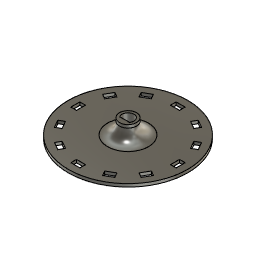
sterivex vortex adapter plate fusion360 (Autodesk Fusion 360 archive; units mm, degrees)
design "Untitled" references "jeej fixed mesh"
Autodesk Fusion 360 part; units mm, degrees
sketch "Sketch3" plane through (0, 0, 0) normal (0, 0, 1) x (1, 0, 0)
  circle A0 centre (0, 0) radius 80
  dimension "d8" = 160
  constraint coincident A0.centre origin
  measures "d8" diameter of A0
extrude "Extrude3" add sketch "Sketch3" along normal blind 4 makes body 1
sketch "Sketch4" plane through (0, 0, 4) normal (0, 0, 1) x (-1, 0, 0)
  circle A0 centre (0, 0) radius 80
  line L0 (0, 0) -> (0, -80) construction
  line L1 (0, -80) -> (0, -82) construction
  line L2 (0, -82) -> (0, -78) construction
  line L3 (6, -62.9579) -> (-6, -62.9579)
  line L4 (-6, -62.9579) -> (-6, -70.4579)
  line L5 (-6, -70.4579) -> (6, -70.4579)
  line L6 (6, -70.4579) -> (6, -62.9579)
  line L7 (6, -62.9579) -> (-6, -70.4579) construction
  line L8 (-6, -62.9579) -> (6, -70.4579) construction
  line L9 (30.0328, -64.0183) -> (40.4251, -58.0183)
  line L10 (36.6751, -51.5231) -> (30.0328, -64.0183) construction
  line L11 (36.6751, -51.5231) -> (26.2828, -57.5231)
  line L12 (40.4251, -58.0183) -> (36.6751, -51.5231)
  line L13 (26.2828, -57.5231) -> (30.0328, -64.0183)
  line L14 (26.2828, -57.5231) -> (40.4251, -58.0183) construction
  line L15 (58.0183, -40.4251) -> (64.0183, -30.0328)
  line L16 (57.5231, -26.2828) -> (58.0183, -40.4251) construction
  line L17 (57.5231, -26.2828) -> (51.5231, -36.6751)
  line L18 (64.0183, -30.0328) -> (57.5231, -26.2828)
  line L19 (51.5231, -36.6751) -> (58.0183, -40.4251)
  line L20 (51.5231, -36.6751) -> (64.0183, -30.0328) construction
  line L21 (70.4579, -6) -> (70.4579, 6)
  line L22 (62.9579, 6) -> (70.4579, -6) construction
  line L23 (62.9579, 6) -> (62.9579, -6)
  line L24 (70.4579, 6) -> (62.9579, 6)
  line L25 (62.9579, -6) -> (70.4579, -6)
  line L26 (62.9579, -6) -> (70.4579, 6) construction
  line L27 (64.0183, 30.0328) -> (58.0183, 40.4251)
  line L28 (51.5231, 36.6751) -> (64.0183, 30.0328) construction
  line L29 (51.5231, 36.6751) -> (57.5231, 26.2828)
  line L30 (58.0183, 40.4251) -> (51.5231, 36.6751)
  line L31 (57.5231, 26.2828) -> (64.0183, 30.0328)
  line L32 (57.5231, 26.2828) -> (58.0183, 40.4251) construction
  line L33 (40.4251, 58.0183) -> (30.0328, 64.0183)
  line L34 (26.2828, 57.5231) -> (40.4251, 58.0183) construction
  line L35 (26.2828, 57.5231) -> (36.6751, 51.5231)
  line L36 (30.0328, 64.0183) -> (26.2828, 57.5231)
  line L37 (36.6751, 51.5231) -> (40.4251, 58.0183)
  line L38 (36.6751, 51.5231) -> (30.0328, 64.0183) construction
  line L39 (6, 70.4579) -> (-6, 70.4579)
  line L40 (-6, 62.9579) -> (6, 70.4579) construction
  line L41 (-6, 62.9579) -> (6, 62.9579)
  line L42 (-6, 70.4579) -> (-6, 62.9579)
  line L43 (6, 62.9579) -> (6, 70.4579)
  line L44 (6, 62.9579) -> (-6, 70.4579) construction
  line L45 (-30.0328, 64.0183) -> (-40.4251, 58.0183)
  line L46 (-36.6751, 51.5231) -> (-30.0328, 64.0183) construction
  line L47 (-36.6751, 51.5231) -> (-26.2828, 57.5231)
  line L48 (-40.4251, 58.0183) -> (-36.6751, 51.5231)
  line L49 (-26.2828, 57.5231) -> (-30.0328, 64.0183)
  line L50 (-26.2828, 57.5231) -> (-40.4251, 58.0183) construction
  line L51 (-58.0183, 40.4251) -> (-64.0183, 30.0328)
  line L52 (-57.5231, 26.2828) -> (-58.0183, 40.4251) construction
  line L53 (-57.5231, 26.2828) -> (-51.5231, 36.6751)
  line L54 (-64.0183, 30.0328) -> (-57.5231, 26.2828)
  line L55 (-51.5231, 36.6751) -> (-58.0183, 40.4251)
  line L56 (-51.5231, 36.6751) -> (-64.0183, 30.0328) construction
  line L57 (-70.4579, 6) -> (-70.4579, -6)
  line L58 (-62.9579, -6) -> (-70.4579, 6) construction
  line L59 (-62.9579, -6) -> (-62.9579, 6)
  line L60 (-70.4579, -6) -> (-62.9579, -6)
  line L61 (-62.9579, 6) -> (-70.4579, 6)
  line L62 (-62.9579, 6) -> (-70.4579, -6) construction
  line L63 (-64.0183, -30.0328) -> (-58.0183, -40.4251)
  line L64 (-51.5231, -36.6751) -> (-64.0183, -30.0328) construction
  line L65 (-51.5231, -36.6751) -> (-57.5231, -26.2828)
  line L66 (-58.0183, -40.4251) -> (-51.5231, -36.6751)
  line L67 (-57.5231, -26.2828) -> (-64.0183, -30.0328)
  line L68 (-57.5231, -26.2828) -> (-58.0183, -40.4251) construction
  line L69 (-40.4251, -58.0183) -> (-30.0328, -64.0183)
  line L70 (-26.2828, -57.5231) -> (-40.4251, -58.0183) construction
  line L71 (-26.2828, -57.5231) -> (-36.6751, -51.5231)
  line L72 (-30.0328, -64.0183) -> (-26.2828, -57.5231)
  line L73 (-36.6751, -51.5231) -> (-40.4251, -58.0183)
  line L74 (-36.6751, -51.5231) -> (-30.0328, -64.0183) construction
  point P0 (0, -66.7079)
  point P1 (39, -67.55)
  point P2 (33.3539, -57.7707)
  point P3 (67.55, -39)
  point P4 (57.7707, -33.3539)
  point P5 (78, 0)
  point P6 (66.7079, 0)
  point P7 (67.55, 39)
  point P8 (57.7707, 33.3539)
  point P9 (39, 67.55)
  point P10 (33.3539, 57.7707)
  point P11 (0, 78)
  point P12 (0, 66.7079)
  point P13 (-39, 67.55)
  point P14 (-33.3539, 57.7707)
  point P15 (-67.55, 39)
  point P16 (-57.7707, 33.3539)
  point P17 (-78, 0)
  point P18 (-66.7079, 0)
  point P19 (-67.55, -39)
  point P20 (-57.7707, -33.3539)
  point P21 (-39, -67.55)
  point P22 (-33.3539, -57.7707)
  dimension "d12" = 360
  dimension "d36" = 80
  dimension "d37" = 12
  dimension "d41" = 7.5
  constraint coincident A0.centre L0.start
  constraint coincident A0 L0.end
  constraint vertical L0
  constraint coincident L0 L1.end
  constraint coincident L0 L2.end
  constraint horizontal L3
  constraint perpendicular L3 L4
  constraint parallel L3 L5
  constraint parallel L4 L6
  constraint coincident L7 P0
  constraint coincident L8 P0
  constraint coincident L0 P0
  measures "d36" distance of A0.centre L0.end
  measures "d37" distance of L3.start L3.end
  measures "d41" distance of L3.end L4.end
extrude "Extrude4" cut sketch "Sketch4" against normal blind 16.943 contours L3 L4 L5 L6 | L9 L11 L12 L13 | L15 L17 L18 L19 | L21 L23 L24 L25 | L27 L29 L30 L31 | L33 L35 L36 L37 | L39 L41 L42 L43 | L45 L47 L48 L49 | L51 L53 L54 L55 | L57 L59 L60 L61 | L63 L65 L66 L67 | L69 L71 L72 L73 bodies 1
sketch "Sketch5" plane through (0, 0, 4) normal (0, 0, 1) x (-1, 0, 0)
  line L0 (40.4251, 58.0183) -> (36.6751, 51.5231)
  line L1 (36.6751, 51.5231) -> (26.2828, 57.5231)
  line L2 (26.2828, 57.5231) -> (30.0328, 64.0183)
  line L3 (30.0328, -64.0183) -> (26.2828, -57.5231)
  line L4 (26.2828, -57.5231) -> (36.6751, -51.5231)
  line L5 (36.6751, -51.5231) -> (40.4251, -58.0183)
  line L6 (-70.4579, 6) -> (-62.9579, 6)
  line L7 (-62.9579, 6) -> (-62.9579, -6)
  line L8 (-62.9579, -6) -> (-70.4579, -6)
  line L9 (-64.0183, -30.0328) -> (-57.5231, -26.2828)
  line L10 (-57.5231, -26.2828) -> (-51.5231, -36.6751)
  line L11 (-51.5231, -36.6751) -> (-58.0183, -40.4251)
  line L12 (58.0183, -40.4251) -> (51.5231, -36.6751)
  line L13 (51.5231, -36.6751) -> (57.5231, -26.2828)
  line L14 (57.5231, -26.2828) -> (64.0183, -30.0328)
  line L15 (6, 70.4579) -> (6, 62.9579)
  line L16 (6, 62.9579) -> (-6, 62.9579)
  line L17 (-6, 62.9579) -> (-6, 70.4579)
  line L18 (64.0183, 30.0328) -> (57.5231, 26.2828)
  line L19 (57.5231, 26.2828) -> (51.5231, 36.6751)
  line L20 (51.5231, 36.6751) -> (58.0183, 40.4251)
  line L21 (-6, -62.9579) -> (6, -62.9579)
  line L22 (6, -62.9579) -> (6, -70.4579)
  line L23 (-6, -70.4579) -> (-6, -62.9579)
  line L24 (-58.0183, 40.4251) -> (-51.5231, 36.6751)
  line L25 (-51.5231, 36.6751) -> (-57.5231, 26.2828)
  line L26 (-57.5231, 26.2828) -> (-64.0183, 30.0328)
  line L27 (-40.4251, -58.0183) -> (-36.6751, -51.5231)
  line L28 (-36.6751, -51.5231) -> (-26.2828, -57.5231)
  line L29 (-26.2828, -57.5231) -> (-30.0328, -64.0183)
  line L30 (70.4579, -6) -> (62.9579, -6)
  line L31 (62.9579, -6) -> (62.9579, 6)
  line L32 (62.9579, 6) -> (70.4579, 6)
  line L33 (-30.0328, 64.0183) -> (-26.2828, 57.5231)
  line L34 (-26.2828, 57.5231) -> (-36.6751, 51.5231)
  line L35 (-36.6751, 51.5231) -> (-40.4251, 58.0183)
  circle A0 centre (0, 0) radius 11.5
  line L36 (30.0328, 64.0183) -> (40.4251, 58.0183)
  line L37 (40.4251, -58.0183) -> (30.0328, -64.0183)
  line L38 (-70.4579, -6) -> (-70.4579, 6)
  line L39 (-58.0183, -40.4251) -> (-64.0183, -30.0328)
  line L40 (64.0183, -30.0328) -> (58.0183, -40.4251)
  line L41 (-6, 70.4579) -> (6, 70.4579)
  line L42 (58.0183, 40.4251) -> (64.0183, 30.0328)
  line L43 (6, -70.4579) -> (-6, -70.4579)
  line L44 (-64.0183, 30.0328) -> (-58.0183, 40.4251)
  line L45 (-30.0328, -64.0183) -> (-40.4251, -58.0183)
  line L46 (70.4579, 6) -> (70.4579, -6)
  line L47 (-40.4251, 58.0183) -> (-30.0328, 64.0183)
  circle A1 centre (0, 0) radius 80
  dimension "d15" = 23
  constraint coincident A0.centre A1.centre
  measures "d15" diameter of A0
extrude "Extrude5" add sketch "Sketch5" along normal blind 20 contours A0 bodies 1
fillet "Fillet1" radius 15.9369 1 edges at (10.7218, -4.1586, 4) on bodies 1
sketch "Sketch6" plane through (0, 0, 24) normal (0, 0, 1) x (-1, 0, 0)
  circle A0 centre (0, 0) radius 8
  line L0 (0, -8) -> (0, 4.5)
  line L1 (0, 4.5) -> (-6.6144, 4.5)
  line L2 (0, 4.5) -> (6.6144, 4.5)
  circle A1 centre (0, 0) radius 11.5
  dimension "d20" = 16
  dimension "d42" = 12.5
  dimension "d43" = 23
  constraint coincident A0.centre A1.centre
  constraint coincident A0 L0.start
  constraint vertical L0
  constraint coincident A0 L1.end
  constraint perpendicular L0 L1
  constraint coincident A0 L2.end
  constraint perpendicular L0 L2
  measures "d20" diameter of A0
  measures "d42" distance of L0.start L0.end
  measures "d43" diameter of A1
extrude "Extrude6" cut sketch "Sketch6" against normal blind 15 contours A0 L0 L2 | A0 L0 L1 bodies 1
copy_body "Body->Comp1" bodies 1 removing the originals makes body 2 in component "Component"
sketch "Sketch1" plane through (0, 62.9579, 0) normal (0, 1, 0) x (-1, 0, 0) in component "Component'"
  line L0 (-6, 0) -> (6, 0)
  line L1 (6, 0) -> (6, 4)
  line L2 (6, 4) -> (-6, 4)
  line L3 (-6, 4) -> (-6, 0)
  line L4 (7, 5) -> (5.7531, 5)
  line L5 (5.7531, 5) -> (5.7531, -0.9021)
  line L6 (7, 5) -> (5, 10)
  line L7 (5, 10) -> (1.6146, 10)
  line L8 (1.6146, 10) -> (0.5203, 0)
  line L9 (0.5203, 0) -> (0, 0)
  line L10 (0, -0.7) -> (0, 1.4)
  line L11 (-0.5203, 0) -> (0, 0)
  line L12 (-1.6146, 10) -> (-0.5203, 0)
  line L13 (-5.7531, 5) -> (-5.7531, -0.9021)
  line L14 (-7, 5) -> (-5.7531, 5)
  line L15 (-7, 5) -> (-5, 10)
  line L16 (-5, 10) -> (-1.6146, 10)
  circle A0 centre (0, -10.2579) radius 7.375
  line L17 (5.7531, -0.9021) -> (7.2493, -8.9021)
  line L18 (-5.7531, -0.9021) -> (-7.2493, -8.9021)
  circle A1 centre (0, -10.2579) radius 9.5
  line L19 (0, -10.2579) -> (5.5, -10.2579)
  line L20 (5.5, -10.2579) -> (5.5, -18.0039)
  line L21 (0, -10.2579) -> (-5.5, -10.2579)
  line L22 (-5.5, -10.2579) -> (-5.5, -18.0039)
  line L23 (-6.1484, -3.0159) -> (6.1484, -3.0159)
  line L24 (6.1484, -3.0159) -> (6.1484, -0.5288)
  line L25 (6.1484, -0.5288) -> (-6.1484, -0.5288)
  line L26 (-6.1484, -0.5288) -> (-6.1484, -3.0159)
  line L27 (-0.7382, 1.9909) -> (0.7382, 1.9909)
  line L28 (-7.2493, -0.5288) -> (7.2493, -0.5288)
  line L29 (7.2493, -0.5288) -> (7.2493, -4.1181)
  line L30 (7.2493, -4.1181) -> (-7.2493, -4.1181)
  line L31 (-7.2493, -4.1181) -> (-7.2493, -0.5288)
  dimension "d25" = 8
  dimension "d27" = 19
  dimension "d28" = 5.5
  dimension "d29" = 5.5
  dimension "d38" = 14.75
  dimension "d48" = 1.2469
  constraint horizontal L4
  constraint perpendicular L0 L5
  constraint perpendicular L5 L7
  constraint coincident L0 L8.end
  constraint coincident L9.end L11.end
  constraint perpendicular L9 L10
  constraint symmetric L4.start L10 L14.start
  constraint symmetric L4.end L10 L13.start
  constraint symmetric L5.end L10 L13.end
  constraint symmetric L6.end L10 L15.end
  constraint symmetric L7.end L10 L12.start
  constraint symmetric L8.end L10 L11.start
  constraint symmetric L9.end L10 L11.end
  constraint coincident A0 L17.end
  constraint tangent A0 L17
  constraint coincident A0 L18.end
  constraint tangent A0 L18
  constraint equal L17 L18
  constraint concentric A0 A1
  constraint coincident A0.centre A1.centre
  constraint horizontal L19
  constraint coincident A1 L20.end
  constraint perpendicular L19 L20
  constraint perpendicular L20 L21
  constraint coincident A1 L22.end
  constraint perpendicular L21 L22
  constraint horizontal L23
  constraint vertical L24
  constraint horizontal L25
  constraint vertical L26
  constraint coincident A1 L23.start
  constraint coincident L18 L23.start
  constraint coincident A1 L23.end
  constraint coincident L12 L27.start
  constraint coincident L8 L27.end
  constraint parallel L14 L27
  constraint horizontal L28
  constraint vertical L29
  constraint horizontal L30
  constraint vertical L31
  constraint coincident A1 L29.end
  measures "d25" vertical distance of L5.end L17.end
  measures "d27" diameter of A1
  measures "d28" distance of A0.centre L21.end
  measures "d29" distance of A0.centre L19.end
  measures "d38" diameter of A0
  measures "d48" distance of L4.start L4.end
extrude "Extrude1" add sketch "Sketch1" along normal blind 7 separate body contours L0 L8 L9 L11 L12 L27 | L0 L10 L11 L13 L25 L28 | L0 L2 L12 L13 | L0 L5 L9 L10 L25 L28 | L0 L2 L5 L8 | L5 L13 L17 L18 A1 L25 L28 | L2 L12 L13 L14 L15 L16 | L13 L18 L25 L26 L28 | L5 L17 L24 L25 L28 | A1 L26 L28 L31 | L2 L4 L5 L6 L7 L8 | A1 L24 L28 L29 | A0 L18 L23 L30 | L18 A1 L30 | A0 A1 L23 | L17 A1 L30 | A0 L17 L23 L30 | A0 L18 L30 | A0 L18 A1 L22 L30 | A0 L17 A1 L20 L30 | A0 L17 L30 makes body 3 in component "Component'"
fillet "Fillet1'" radius 1 2 edges at (-7, 66.4579, 5) (7, 66.4579, 5) on bodies 3 in component "Component'"
fillet "Fillet2" radius 1 2 edges at (-5.5, 66.4579, -18.0039) (5.5, 66.4579, -18.0039) on bodies 3 in component "Component'"
component_pattern "component pattern" in component "Component"
sketch "Sketch7" plane through (0, 0, 0) normal (0, 0, -1) x (1, 0, 0)
  line L0 (-40.4251, 58.0183) -> (-30.0328, 64.0183)
  line L1 (-30.0328, 64.0183) -> (-26.2828, 57.5231)
  line L2 (-26.2828, 57.5231) -> (-36.6751, 51.5231)
  line L3 (-36.6751, 51.5231) -> (-40.4251, 58.0183)
  line L4 (-30.0328, -64.0183) -> (-40.4251, -58.0183)
  line L5 (-40.4251, -58.0183) -> (-36.6751, -51.5231)
  line L6 (-36.6751, -51.5231) -> (-26.2828, -57.5231)
  line L7 (-26.2828, -57.5231) -> (-30.0328, -64.0183)
  line L8 (70.4579, 6) -> (70.4579, -6)
  line L9 (70.4579, -6) -> (62.9579, -6)
  line L10 (62.9579, -6) -> (62.9579, 6)
  line L11 (62.9579, 6) -> (70.4579, 6)
  line L12 (64.0183, -30.0328) -> (58.0183, -40.4251)
  line L13 (58.0183, -40.4251) -> (51.5231, -36.6751)
  line L14 (51.5231, -36.6751) -> (57.5231, -26.2828)
  line L15 (57.5231, -26.2828) -> (64.0183, -30.0328)
  line L16 (-58.0183, -40.4251) -> (-64.0183, -30.0328)
  line L17 (-64.0183, -30.0328) -> (-57.5231, -26.2828)
  line L18 (-57.5231, -26.2828) -> (-51.5231, -36.6751)
  line L19 (-51.5231, -36.6751) -> (-58.0183, -40.4251)
  line L20 (-6, 70.4579) -> (6, 70.4579)
  line L21 (6, 70.4579) -> (6, 62.9579)
  line L22 (6, 62.9579) -> (-6, 62.9579)
  line L23 (-6, 62.9579) -> (-6, 70.4579)
  line L24 (-64.0183, 30.0328) -> (-58.0183, 40.4251)
  line L25 (-58.0183, 40.4251) -> (-51.5231, 36.6751)
  line L26 (-51.5231, 36.6751) -> (-57.5231, 26.2828)
  line L27 (-57.5231, 26.2828) -> (-64.0183, 30.0328)
  line L28 (-6, -62.9579) -> (6, -62.9579)
  line L29 (6, -62.9579) -> (6, -70.4579)
  line L30 (6, -70.4579) -> (-6, -70.4579)
  line L31 (-6, -70.4579) -> (-6, -62.9579)
  line L32 (58.0183, 40.4251) -> (64.0183, 30.0328)
  line L33 (64.0183, 30.0328) -> (57.5231, 26.2828)
  line L34 (57.5231, 26.2828) -> (51.5231, 36.6751)
  line L35 (51.5231, 36.6751) -> (58.0183, 40.4251)
  line L36 (40.4251, -58.0183) -> (30.0328, -64.0183)
  line L37 (30.0328, -64.0183) -> (26.2828, -57.5231)
  line L38 (26.2828, -57.5231) -> (36.6751, -51.5231)
  line L39 (36.6751, -51.5231) -> (40.4251, -58.0183)
  line L40 (-70.4579, -6) -> (-70.4579, 6)
  line L41 (-70.4579, 6) -> (-62.9579, 6)
  line L42 (-62.9579, 6) -> (-62.9579, -6)
  line L43 (-62.9579, -6) -> (-70.4579, -6)
  line L44 (30.0328, 64.0183) -> (40.4251, 58.0183)
  line L45 (40.4251, 58.0183) -> (36.6751, 51.5231)
  line L46 (36.6751, 51.5231) -> (26.2828, 57.5231)
  line L47 (26.2828, 57.5231) -> (30.0328, 64.0183)
  circle A0 centre (0, 0) radius 80
  line L48 (3.75, -3.75) -> (-3.75, -3.75)
  line L49 (-3.75, -3.75) -> (-3.75, 3.75)
  line L50 (-3.75, 3.75) -> (3.75, 3.75)
  line L51 (3.75, 3.75) -> (3.75, -3.75)
  line L52 (3.75, -3.75) -> (-3.75, 3.75) construction
  line L53 (-3.75, -3.75) -> (3.75, 3.75) construction
  dimension "d44" = 7.5
  dimension "d45" = 7.5
  constraint horizontal L48
  constraint perpendicular L48 L49
  constraint parallel L48 L50
  constraint parallel L49 L51
  constraint coincident L52 A0.centre
  constraint coincident L53 A0.centre
  constraint coincident A0.centre origin
  measures "d44" distance of L49.end L50.end
  measures "d45" distance of L48.end L49.end
extrude "Extrude1'" cut sketch "Sketch7" against normal blind 5 contours L48 L49 L50 L51 bodies 2 in component "Component"
component "Component" placed x (1, 0, 0) y (0, 1, 0) z (0, 0, 1) at (0, 0, 0)
component "Component'" placed x (1, 0, 0) y (0, 1, 0) z (0, 0, 1) at (0, 0, 0) in component "Component"
component "Component'" placed x (0.866025, 0.5, 0) y (-0.5, 0.866025, 0) z (0, 0, 1) at (0, 0, 0) in component "Component"
component "Component'" placed x (0.5, 0.866025, 0) y (-0.866025, 0.5, 0) z (0, 0, 1) at (0, 0, 0) in component "Component"
component "Component'" placed x (0, 1, 0) y (-1, 0, 0) z (0, 0, 1) at (0, 0, 0) in component "Component"
component "Component'" placed x (-0.5, 0.866025, 0) y (-0.866025, -0.5, 0) z (0, 0, 1) at (0, 0, 0) in component "Component"
component "Component'" placed x (-0.866025, 0.5, 0) y (-0.5, -0.866025, 0) z (0, 0, 1) at (0, 0, 0) in component "Component"
component "Component'" placed x (-1, 0, 0) y (0, -1, 0) z (0, 0, 1) at (0, 0, 0) in component "Component"
component "Component'" placed x (-0.866025, -0.5, 0) y (0.5, -0.866025, 0) z (0, 0, 1) at (0, 0, 0) in component "Component"
component "Component'" placed x (-0.5, -0.866025, 0) y (0.866025, -0.5, 0) z (0, 0, 1) at (0, 0, 0) in component "Component"
component "Component'" placed x (0, -1, 0) y (1, 0, 0) z (0, 0, 1) at (0, 0, 0) in component "Component"
component "Component'" placed x (0.5, -0.866025, 0) y (0.866025, 0.5, 0) z (0, 0, 1) at (0, 0, 0) in component "Component"
component "Component'" placed x (0.866025, -0.5, 0) y (0.5, 0.866025, 0) z (0, 0, 1) at (0, 0, 0) in component "Component"
